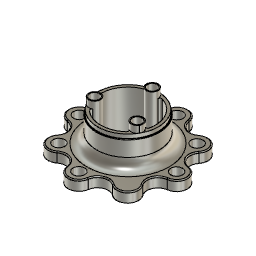
drive flange v1 (Autodesk Fusion 360 design; units mm, degrees)
Autodesk Fusion 360 part; units mm, degrees
sketch "Sketch1" plane through (0, 0, 0) normal (0, 0, 1) x (1, 0, 0)
  circle A0 centre (0, 0) radius 50 construction
  circle A1 centre (0.2426, 49.9994) radius 6
  circle A2 centre (-35.1834, 35.5265) radius 6
  circle A3 centre (-49.9994, 0.2426) radius 6
  circle A4 centre (-35.5265, -35.1834) radius 6
  circle A5 centre (-0.2426, -49.9994) radius 6
  circle A6 centre (49.9994, -0.2426) radius 6
  circle A7 centre (35.5265, 35.1834) radius 6
  arc A8 (11.1653, 51.3007) -> (28.8073, 43.8927) centre (22.0881, 52.6021) ccw
  arc A9 (44.1702, 28.38) -> (51.4067, 10.667) centre (52.8139, 21.5766) ccw
  arc A10 (51.3007, -11.1653) -> (43.8927, -28.8073) centre (52.6021, -22.0881) ccw
  arc A11 (28.38, -44.1702) -> (10.667, -51.4067) centre (21.5766, -52.8139) ccw
  arc A12 (-11.1653, -51.3007) -> (-28.8073, -43.8927) centre (-22.0881, -52.6021) ccw
  arc A13 (-44.1702, -28.38) -> (-51.4067, -10.667) centre (-52.8139, -21.5766) ccw
  arc A14 (-51.3007, 11.1653) -> (-43.8927, 28.8073) centre (-52.6021, 22.0881) ccw
  arc A15 (-28.38, 44.1702) -> (-10.667, 51.4067) centre (-21.5766, 52.8139) ccw
  arc A16 (-26.5636, 42.3601) -> (-42.1003, 26.9733) centre (-35.1834, 35.5265) ccw
  arc A17 (11.1698, 48.7364) -> (-10.6964, 48.8425) centre (0.2426, 49.9994) ccw
  arc A18 (42.3601, 26.5636) -> (26.9733, 42.1003) centre (35.5265, 35.1834) ccw
  arc A19 (48.7364, -11.1698) -> (48.8425, 10.6964) centre (49.9994, -0.2426) ccw
  arc A20 (26.5636, -42.3601) -> (42.1003, -26.9733) centre (35.1834, -35.5265) ccw
  arc A21 (30.6746, -39.4851) -> (39.1856, -31.0563) centre (35.1834, -35.5265) ccw
  arc A22 (-11.1698, -48.7364) -> (10.6964, -48.8425) centre (-0.2426, -49.9994) ccw
  arc A23 (-42.3601, -26.5636) -> (-26.9733, -42.1003) centre (-35.5265, -35.1834) ccw
  arc A24 (-48.7364, 11.1698) -> (-48.8425, -10.6964) centre (-49.9994, 0.2426) ccw
  dimension "d1" = 100
  dimension "d2" = 22
  dimension "d3" = 12
  dimension "d6" = 22
  constraint coincident A0.centre origin
  constraint coincident A0 A1.centre
  constraint concentric A1 A17
  constraint tangent A15 A17
  constraint tangent A15 A16
  constraint coincident A8.end A18
  constraint coincident A8.start A17
  constraint coincident A9.end A19
  constraint coincident A9.start A18
  constraint coincident A10.end A20
  constraint coincident A10.start A19
  constraint coincident A11.end A22
  constraint coincident A11.start A20
  constraint coincident A12.end A23
  constraint coincident A12.start A22
  constraint coincident A13.end A24
  constraint coincident A13.start A23
  constraint coincident A14.end A16
  constraint coincident A14.start A24
  constraint coincident A15.end A17
  constraint coincident A15.start A16
  constraint coincident A0 A16.end
  constraint coincident A0 A16.start
  constraint coincident A0 A17.end
  constraint coincident A0 A17.start
  constraint coincident A0 A18.end
  constraint coincident A0 A18.start
  constraint coincident A0 A19.end
  constraint coincident A0 A19.start
  constraint coincident A0 A20.end
  constraint coincident A0 A20.start
  constraint coincident A0 A21.end
  constraint coincident A0 A21.start
  constraint coincident A0 A22.end
  constraint coincident A0 A22.start
  constraint coincident A0 A23.end
  constraint coincident A0 A23.start
  constraint coincident A0 A24.end
  constraint coincident A0 A24.start
  measures "d1" diameter of A0
  measures "d2" diameter of A17
  measures "d3" diameter of A1
  measures "d6" diameter of A15
extrude "Extrude1" add sketch "Sketch1" along normal blind 10
sketch "Sketch2" plane through (0, 0, 10) normal (0, 0, 1) x (-1, 0, 0)
  circle A0 centre (0.2426, 49.9994) radius 6
  circle A1 centre (-0.2426, -49.9994) radius 6
  circle A2 centre (-49.9994, 0.2426) radius 6
  circle A3 centre (-35.5265, -35.1834) radius 6
  circle A4 centre (49.9994, -0.2426) radius 6
  circle A5 centre (35.5265, 35.1834) radius 6
  circle A6 centre (35.1834, -35.5265) radius 6
  arc A7 (44.1702, 28.38) -> (28.8073, 43.8927) centre (35.5265, 35.1834) ccw
  arc A8 (11.1653, 51.3007) -> (28.8073, 43.8927) centre (22.0881, 52.6021) ccw
  arc A9 (11.1653, 51.3007) -> (-10.667, 51.4067) centre (0.2426, 49.9994) ccw
  arc A10 (-28.38, 44.1702) -> (-10.667, 51.4067) centre (-21.5766, 52.8139) ccw
  arc A11 (-28.38, 44.1702) -> (-43.8927, 28.8073) centre (-35.1834, 35.5265) ccw
  arc A12 (-51.3007, 11.1653) -> (-43.8927, 28.8073) centre (-52.6021, 22.0881) ccw
  arc A13 (-51.3007, 11.1653) -> (-51.4067, -10.667) centre (-49.9994, 0.2426) ccw
  arc A14 (-44.1702, -28.38) -> (-51.4067, -10.667) centre (-52.8139, -21.5766) ccw
  arc A15 (-44.1702, -28.38) -> (-28.8073, -43.8927) centre (-35.5265, -35.1834) ccw
  arc A16 (-11.1653, -51.3007) -> (-28.8073, -43.8927) centre (-22.0881, -52.6021) ccw
  arc A17 (-11.1653, -51.3007) -> (10.667, -51.4067) centre (-0.2426, -49.9994) ccw
  arc A18 (28.38, -44.1702) -> (10.667, -51.4067) centre (21.5766, -52.8139) ccw
  arc A19 (28.38, -44.1702) -> (43.8927, -28.8073) centre (35.1834, -35.5265) ccw
  arc A20 (51.3007, -11.1653) -> (43.8927, -28.8073) centre (52.6021, -22.0881) ccw
  arc A21 (51.3007, -11.1653) -> (51.4067, 10.667) centre (49.9994, -0.2426) ccw
  arc A22 (44.1702, 28.38) -> (51.4067, 10.667) centre (52.8139, 21.5766) ccw
  circle A23 centre (0, 0) radius 32
  dimension "d11" = 64
  constraint coincident A23.centre origin
  measures "d11" diameter of A23
extrude "Extrude2" add sketch "Sketch2" along normal blind 26 contours A23
sketch "Sketch3" plane through (0, 0, 36) normal (0, 0, 1) x (-1, 0, 0)
  circle A0 centre (0, 0) radius 32
  circle A1 centre (0, 0) radius 31
  dimension "d14" = 62
  constraint coincident A0.centre A1.centre
  measures "d14" diameter of A1
extrude "Extrude3" add sketch "Sketch3" along normal blind 4 contours A1
fillet "Fillet1" radius 1 16 edges at (42.4599, -17.8293, 10) (60.9993, -0.2959, 10) (42.6309, 17.4165, 10) (43.3423, 42.9237, 10) (17.8293, 42.4599, 10) (0.2959, 60.9993, 10) (-17.4165, 42.6309, 10) (-42.9237, 43.3423, 10) (-42.4599, 17.8293, 10) (-60.9993, 0.2959, 10) (-42.6309, -17.4165, 10) (-43.3423, -42.9237, 10) (-17.8293, -42.4599, 10) (-0.2959, -60.9993, 10) (17.4165, -42.6309, 10) (42.9237, -43.3423, 10)
fillet "Fillet2" radius 10 1 edges at (29.8345, -11.5717, 10)
fillet "Fillet3" radius 0.5 1 edges at (29.8345, 11.5717, 36)
sketch "Sketch4" plane through (0, 0, 40) normal (0, 0, 1) x (-1, 0, 0)
  circle A0 centre (0, 0) radius 31
  circle A1 centre (0.1426, -25) radius 6
  circle A2 centre (0.1426, -25) radius 5
  circle A3 centre (21.5793, 12.6235) radius 5
  circle A4 centre (21.5793, 12.6235) radius 6
  circle A5 centre (-21.7219, 12.3765) radius 5
  circle A6 centre (-21.7219, 12.3765) radius 6
  arc A7 (-26.5682, 8.8391) -> (-5.316, -27.4907) centre (0, 0) ccw
  arc A8 (5.6292, -27.4283) -> (26.4657, 9.1416) centre (0, 0) ccw
  arc A9 (20.939, 18.5892) -> (-21.1497, 18.3492) centre (0, 0) ccw
  dimension "d23" = 12
  dimension "d24" = 10
  dimension "d25" = 25
  dimension "d28" = 56
  constraint concentric A1 A2
  constraint coincident A0.centre A7.centre
  constraint coincident A1 A8.start
  constraint coincident A1 A7.end
  constraint coincident A6 A7.start
  constraint concentric A7 A8
  constraint coincident A6 A9.end
  constraint coincident A4 A8.end
  constraint concentric A8 A9
  constraint coincident A4 A9.start
  measures "d23" diameter of A1
  measures "d24" diameter of A2
  measures "d25" vertical distance of A0.centre A1.centre
  measures "d28" diameter of A8
extrude "Extrude4" cut sketch "Sketch4" against normal blind 65.408 contours A1 A4 A6 A7 A8 A9
extrude "Extrude5" add sketch "Sketch4" along normal blind 7 contours A4 | A1 | A6
extrude "Extrude6" cut sketch "Sketch4" against normal blind 86.44 contours A2 | A3 | A5
fillet "Fillet4" radius 2 6 edges at (5.316, 27.4907, 20) (-5.6292, 27.4283, 20) (-20.939, -18.5892, 20) (-26.4657, -9.1416, 20) (26.5682, -8.8391, 20) (21.1497, -18.3492, 20)
